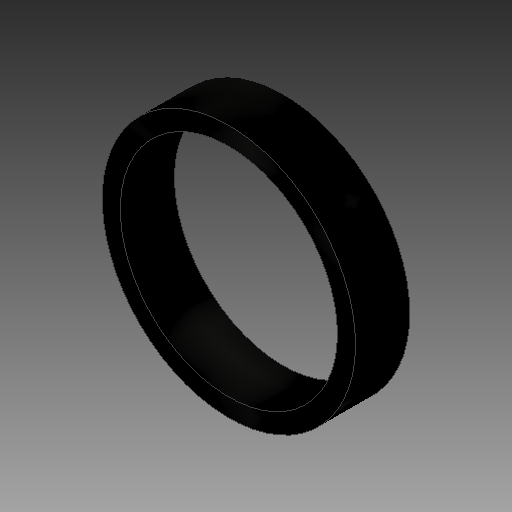
# Autodesk Inventor part: オイレス121403
Saved by Autodesk Inventor 2019 (Build 230136000, 136)
## iProperties
Part Number: オイレス121403
Material: アセタール樹脂、黒
Document SubType Name: Modeling
Designer: 雪村
Density: 1.425 g/cm^3
Appearance: 滑らか - 黒
Mass: 0.174594 g
Surface Area: 3.26726 cm^2
Volume: 0.122522 cm^3
Author: 雪村
Autodesk Inventor part; units mm, degrees
ref_plane "YZ Plane" through (0, 0, 0) normal (1, 0, 0) x (0, 1, 0)
ref_plane "XZ Plane" through (0, 0, 0) normal (0, 1, 0) x (-1, 0, 0)
ref_plane "XY Plane" through (0, 0, 0) normal (0, 0, 1) x (1, 0, 0)
sketch "スケッチ1" plane through (0, 0, 0) normal (0, 0, 1) x (1, 0, 0)
  circle A0 centre (0, 0) radius 6
  circle A1 centre (0, 0) radius 7
  dimension "d0" = 12
  dimension "d1" = 14
  constraints: 2 centre point, 2 coincident
  measures "d0" diameter of A0
  measures "d1" diameter of A1
extrude "押し出し1" add sketch "スケッチ1" along normal blind 3
